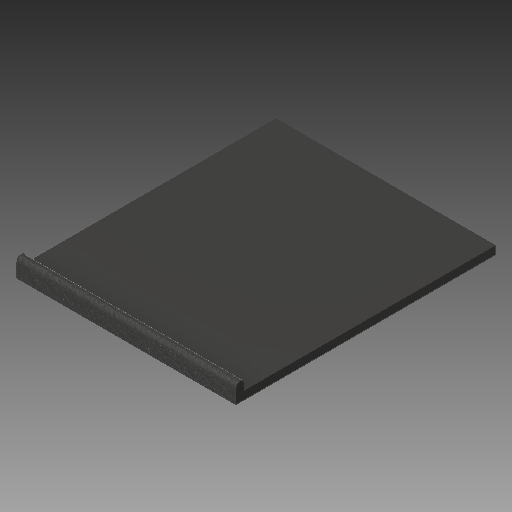
# Autodesk Inventor part: WYSUWANY PLASTIK
Saved by Autodesk Inventor 2017 SP1 (Build 210196100, 196)
## iProperties
Created: 2021-03-07
Part Number: WYSUWANY PLASTIK
Material: Tworzywo sztuczne, nieprzezroczyste czarne
Document SubType Name: Modeling
Designer: Administrator
Density: 0.952 g/cm^3
Appearance: Gładkie - czarne
Author: Administrator
Autodesk Inventor part; units mm, degrees
ref_plane "YZ Plane" through (0, 0, 0) normal (1, 0, 0) x (0, 1, 0)
ref_plane "XZ Plane" through (0, 0, 0) normal (0, 1, 0) x (-1, 0, 0)
ref_plane "XY Plane" through (0, 0, 0) normal (0, 0, 1) x (1, 0, 0)
sketch "Szkic1" plane through (0, 0, 0) normal (0, 0, 1) x (1, 0, 0)
  line L0 (57.7, 0) -> (5.3, 0)
  line L1 (5.3, -4.3965) -> (5.3, 0)
  line L2 (57.7, -4.3965) -> (57.7, 0)
  line L3 (5.3, -4.3965) -> (57.7, -4.3965)
  constraints: 8 end point, 1 horizontal, 1 perpendicular
extrude "Wyciągnięcie proste1" add sketch "Szkic1" against normal blind 2
fillet "Zaokrąglenie1" radius 1 2 edges at (31.5, 0, 0) (31.5, 0, -2) curvature continuous yes
sketch "Szkic2" plane through (0, 0, -2) normal (0, 0, -1) x (-1, 0, 0)
  line L0 (-57.7, -2.3965) -> (-5.3, -2.3965)
  line L1 (-5.3, -2.3965) -> (-5.3, -4.3965)
  line L2 (-5.3, -4.3965) -> (-57.7, -4.3965)
  line L3 (-57.7, -4.3965) -> (-57.7, -2.3965)
  constraints: 8 end point, 2 parallel, 1 horizontal, 1 perpendicular
extrude "Wyciągnięcie proste2" add sketch "Szkic2" along normal blind 60
